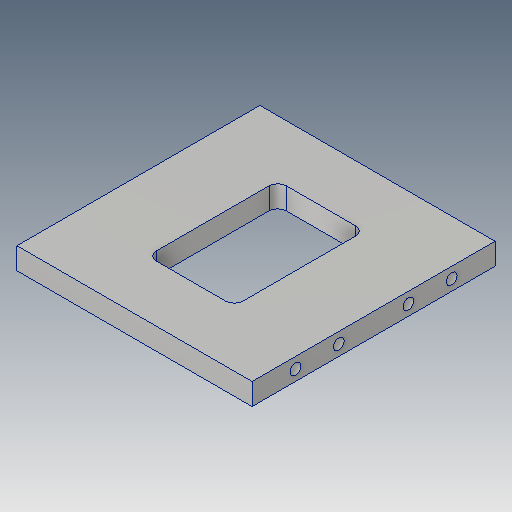
# Autodesk Inventor part: J1J2_Bottom
Saved by Autodesk Inventor 2020.5 (Build 245400000, 400)
## iProperties
Created: 2021-07-07
Part Number: J1J2_Bottom
Material: 알루미늄 6061
Document SubType Name: Modeling
Designer: user
Density: 2.7 g/cm^3
Appearance: 알루미늄 - 평지
Mass: 32.0733 g
Surface Area: 69.6475 cm^2
Volume: 11.879 cm^3
Author: user
Autodesk Inventor part; units mm, degrees
ref_plane "YZ Plane" through (0, 0, 0) normal (1, 0, 0) x (0, 1, 0)
ref_plane "XZ Plane" through (0, 0, 0) normal (0, 1, 0) x (-1, 0, 0)
ref_plane "XY Plane" through (0, 0, 0) normal (0, 0, 1) x (1, 0, 0)
sketch "스케치1" plane through (0, 0, 0) normal (0, 1, 0) x (-1, 0, 0)
  line L0 (27.1, 28) -> (-27.1, 28)
  line L1 (-27.1, 28) -> (-27.1, -28)
  line L2 (-27.1, -28) -> (27.1, -28)
  line L3 (27.1, -28) -> (27.1, 28)
  point P0 (0, 0)
  dimension "d0" = 54.2
  dimension "d1" = 56
  dimension "d2" = 27.1
  dimension "d3" = 28
  constraints: 8 end point, 2 parallel, 1 horizontal, 1 perpendicular
  measures "d0" distance of L2.end L1.end
  measures "d1" distance of L1.end L0.end
  measures "d2" distance from line of L3 point (0, 0)
  measures "d3" distance from line of L0 point (0, 0)
extrude "돌출1" add sketch "스케치1" along normal blind 5
sketch "스케치5" plane through (27.1, 0, 28) normal (1, 0, 0) x (0, 0, -1)
  line L0 (0, 0) -> (56, 0) projected
  line L1 (56, 0) -> (56, 5) projected
  line L2 (0, 5) -> (56, 5) projected
  line L3 (0, 0) -> (0, 5) projected
  circle A0 centre (10, 2.5) radius 1.25
  circle A1 centre (20, 2.5) radius 1.25
  circle A2 centre (46, 2.5) radius 1.25
  circle A3 centre (36, 2.5) radius 1.25
  point P0 (28, 0)
  dimension "d16" = 2.5
  dimension "d17" = 2.5
  dimension "d18" = 2.5
  dimension "d19" = 2.5
  dimension "d20" = 2.5
  dimension "d21" = 2.5
  dimension "d22" = 2.5
  dimension "d23" = 2.5
  dimension "d24" = 10
  dimension "d25" = 20
  dimension "d26" = 20
  dimension "d27" = 10
  constraints: 4 centre point
  measures "d16" diameter of A0
  measures "d17" diameter of A1
  measures "d18" diameter of A2
  measures "d19" diameter of A3
  measures "d20" distance from line of L2 A0.centre
  measures "d21" distance from line of L2 A1.centre
  measures "d22" distance from line of L2 A2.centre
  measures "d23" distance from line of L2 A3.centre
  measures "d24" distance from line of L3 A0.centre
  measures "d25" distance from line of L3 A1.centre
  measures "d26" distance from line of L1 A3.centre
  measures "d27" distance from line of L1 A2.centre
extrude "돌출5" cut sketch "스케치5" against normal blind 8 contours A0 | A1 | A2 | A3
sketch "스케치6" plane through (-27.1, 0, -28) normal (-1, 0, 0) x (0, 0, 1)
  circle A0 centre (10, 2.5) radius 1.25 projected
  circle A1 centre (46, 2.5) radius 1.25 projected
  circle A2 centre (36, 2.5) radius 1.25 projected
  circle A3 centre (20, 2.5) radius 1.25 projected
  line L0 (56, 0) -> (0, 0) projected
  line L1 (0, 0) -> (0, 5) projected
  line L2 (56, 5) -> (0, 5) projected
  line L3 (56, 0) -> (56, 5) projected
  point P0 (28, 0)
extrude "돌출6" cut sketch "스케치6" against normal blind 8 contours A0 | A1 | A2 | A3
sketch "스케치7" plane through (0, 5, 0) normal (0, 1, 0) x (1, 0, 0)
  line L0 (-10, 15) -> (10, 15)
  line L1 (10, 15) -> (10, -15)
  line L2 (10, -15) -> (-10, -15)
  line L3 (-10, -15) -> (-10, 15)
  point P0 (0, 0)
  dimension "d32" = 20
  dimension "d33" = 30
  dimension "d34" = 10
  dimension "d35" = 15
  constraints: 8 end point, 2 equal length, 1 horizontal, 1 perpendicular
  measures "d32" distance of L1.end L2.end
  measures "d33" distance of L0.end L1.end
  measures "d34" distance from line of L1 point (0, 0)
  measures "d35" distance from line of L0 point (0, 0)
extrude "돌출7" cut sketch "스케치7" against normal up to surface (5 mm away)
fillet "모깎기1" radius 2 4 edges at (-10, 2.5, -15) (10, 2.5, -15) (-10, 2.5, 15) (10, 2.5, 15)
equation "\"d2\" = 0.5 * d0"
equation "\"d3\" = 0.5 * d1"
equation "\"d34\" = 0.5 * d32"
equation "\"d35\" = 0.5 * d33"
